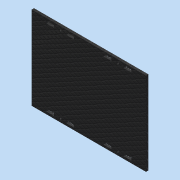
# Autodesk Inventor part: Box Top
Saved by Autodesk Inventor 2013 (Build 170138000, 138)
## iProperties
Created: 2012-12-29
Part Number: Box Top
Material: Generic
Document SubType Name: Modeling
Designer: Administrator
Density: 1 g/cm^3
Author: Administrator
Autodesk Inventor part; units mm, degrees
ref_plane "YZ Plane" through (0, 0, 0) normal (1, 0, 0) x (0, 1, 0)
ref_plane "XZ Plane" through (0, 0, 0) normal (0, 1, 0) x (-1, 0, 0)
ref_plane "XY Plane" through (0, 0, 0) normal (0, 0, 1) x (1, 0, 0)
sketch "Sketch1" plane through (0, 0, 0) normal (0, 0, 1) x (1, 0, 0)
  line L0 (73.3, 53.2739) -> (73.3, -53.4061)
  line L1 (-73.1, -53.4061) -> (-73.1, 53.34)
  line L2 (-73.1, 53.34) -> (-34.8098, 53.34)
  line L3 (36.8493, 53.2398) -> (36.8645, 53.2398)
  line L4 (-34.8098, 53.34) -> (35.3039, 53.34)
  line L5 (38.3039, 53.2739) -> (73.3, 53.2739)
  line L6 (73.3, -53.4061) -> (38.3497, -53.4061)
  circle A0 centre (-36.6002, 48.84) radius 1.525
  line L7 (35.3039, 53.34) -> (38.3039, 53.2739)
  circle A1 centre (36.8039, 48.84) radius 1.525
  line L8 (38.3497, -53.4061) -> (-73.1, -53.4061)
  circle A2 centre (-36.6002, -48.9061) radius 1.525
  circle A3 centre (36.8002, -48.9061) radius 1.525
  line L9 (-44.4252, 50.365) -> (-54.4252, 50.365)
  line L10 (-54.4252, 50.365) -> (-54.4252, 47.365)
  line L11 (-54.4252, 47.365) -> (-44.4252, 47.365)
  line L12 (-44.4252, 47.365) -> (-44.4252, 50.365)
  line L13 (-28.7752, 50.365) -> (-18.7752, 50.365)
  line L14 (-18.7752, 50.365) -> (-18.7752, 47.365)
  line L15 (-18.7752, 47.365) -> (-28.7752, 47.365)
  line L16 (-28.7752, 47.365) -> (-28.7752, 50.365)
  line L17 (28.9789, 50.4163) -> (18.9789, 50.4163)
  line L18 (18.9789, 50.4163) -> (18.9789, 47.3163)
  line L19 (18.9789, 47.3163) -> (28.9789, 47.3163)
  line L20 (28.9789, 47.3163) -> (28.9789, 50.4163)
  line L21 (44.6289, 50.3675) -> (54.6289, 50.3675)
  line L22 (54.6289, 50.3675) -> (54.6289, 47.2675)
  line L23 (54.6289, 47.2675) -> (44.6289, 47.2675)
  line L24 (44.6289, 47.2675) -> (44.6289, 50.3675)
  line L25 (44.6252, -47.3717) -> (54.6252, -47.3717)
  line L26 (54.6252, -47.3717) -> (54.6252, -50.4717)
  line L27 (54.6252, -50.4717) -> (44.6252, -50.4717)
  line L28 (44.6252, -50.4717) -> (44.6252, -47.3717)
  line L29 (28.9752, -47.3717) -> (18.9752, -47.3717)
  line L30 (18.9752, -47.3717) -> (18.9752, -50.4717)
  line L31 (18.9752, -50.4717) -> (28.9752, -50.4717)
  line L32 (28.9752, -50.4717) -> (28.9752, -47.3717)
  line L33 (-28.7752, -47.3535) -> (-18.7752, -47.3535)
  line L34 (-18.7752, -47.3535) -> (-18.7752, -50.4535)
  line L35 (-18.7752, -50.4535) -> (-28.7752, -50.4535)
  line L36 (-28.7752, -50.4535) -> (-28.7752, -47.3535)
  line L37 (-44.4252, -47.3535) -> (-54.4252, -47.3535)
  line L38 (-54.4252, -47.3535) -> (-54.4252, -50.4535)
  line L39 (-54.4252, -50.4535) -> (-44.4252, -50.4535)
  line L40 (-44.4252, -50.4535) -> (-44.4252, -47.3535)
  point P0 (0, 0)
  dimension "d0" = 146.4
  dimension "d1" = 106.68
  dimension "d43" = 3.05
  dimension "d44" = 4.5
  dimension "d45" = 36.4998
  dimension "d47" = 3.05
  dimension "d48" = 36.4961
  dimension "d50" = 3.05
  dimension "d52" = 36.4998
  dimension "d53" = 3.05
  dimension "d54" = 36.4998
  dimension "d58" = 10
  dimension "d59" = 3
  dimension "d60" = 6.3
  dimension "d61" = 10
  dimension "d62" = 3
  dimension "d63" = 6.3
  dimension "d64" = 10
  dimension "d65" = 3.1
  dimension "d66" = 6.3
  dimension "d67" = 10
  dimension "d68" = 3.1
  dimension "d70" = 10
  dimension "d71" = 3.1
  dimension "d73" = 10
  dimension "d74" = 3.1
  dimension "d75" = 6.3
  dimension "d76" = 10
  dimension "d77" = 3.1
  dimension "d79" = 10
  dimension "d80" = 3.1
  dimension "d84" = 6.3
  dimension "d85" = 6.3
  dimension "d86" = 6.3
  dimension "d87" = 6.3
  constraints: 82 end point, 21 parallel, 10 horizontal, 10 perpendicular, 4 centre point, 1 collinear
  measures "d0" distance of L0.end L1.start
  measures "d1" distance of L0.start L0.end
  measures "d43" diameter of A0
  measures "d44" distance from line of L2 A0.centre
  measures "d45" distance from line of L1 A0.centre
  measures "d47" diameter of A1
  measures "d48" distance from line of L0 A1.centre
  measures "d50" diameter of A2
  measures "d52" distance from line of L1 A2.centre
  measures "d53" diameter of A3
  measures "d54" distance from line of L0 A3.centre
  measures "d58" distance of L11.end L10.end
  measures "d59" distance of L10.end L9.end
  measures "d60" distance edge to line of A0 L12
  measures "d61" distance of L14.end L15.end
  measures "d62" distance of L13.end L14.end
  measures "d63" distance edge to line of A0 L16
  measures "d64" distance of L19.end L18.end
  measures "d65" distance of L18.end L17.end
  measures "d66" distance edge to line of A1 L20
  measures "d67" distance of L22.end L23.end
  measures "d68" distance of L21.end L22.end
  measures "d70" distance of L26.end L27.end
  measures "d71" distance of L25.end L26.end
  measures "d73" distance of L31.end L30.end
  measures "d74" distance of L30.end L29.end
  measures "d75" distance edge to line of A3 L32
  measures "d76" distance of L34.end L35.end
  measures "d77" distance of L33.end L34.end
  measures "d79" distance of L39.end L38.end
  measures "d80" distance of L38.end L37.end
  measures "d84" distance edge to line of A1 L24
  measures "d85" distance edge to line of A3 L28
  measures "d86" distance edge to line of A2 L36
  measures "d87" distance edge to line of A2 L40
extrude "Extrusion3" add sketch "Sketch1" along normal blind 3
body "Solid3"
